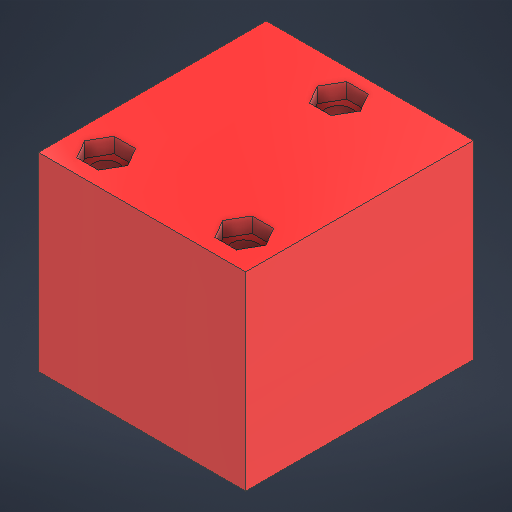
# Autodesk Inventor part: adapter-optical
Saved by Autodesk Inventor 2026.2 (Build 302298000, 298)
## iProperties
Created: 2026-05-22
Part Number: adapter-optical
Material: Generic
Document SubType Name: Modeling
Designer: mayhe
Density: 1 g/cm^3
Appearance: Default
Author: mayhe
Autodesk Inventor part; units mm, degrees
ref_plane "YZ Plane" through (0, 0, 0) normal (1, 0, 0) x (0, 1, 0)
ref_plane "XZ Plane" through (0, 0, 0) normal (0, 1, 0) x (-1, 0, 0)
ref_plane "XY Plane" through (0, 0, 0) normal (0, 0, 1) x (1, 0, 0)
sketch "Sketch1" plane through (0, 0, 0) normal (1, 0, 0) x (0, 1, 0)
  line L0 (13.75, 16.5) -> (-13.75, 16.5)
  line L1 (-13.75, 16.5) -> (-13.75, -16.5)
  line L2 (-13.75, -16.5) -> (13.75, -16.5)
  line L3 (13.75, -16.5) -> (13.75, 16.5)
  line L4 (13.75, 16.5) -> (-13.75, -16.5) construction
  line L5 (-13.75, 16.5) -> (13.75, -16.5) construction
  point P0 (0, 0)
  dimension "d0" = 27.5
  dimension "d1" = 33
  constraints: 12 end point, 2 midpoint, 2 parallel, 1 horizontal, 1 perpendicular
  measures "d0" distance of L2.end L1.end
  measures "d1" distance of L1.end L0.end
extrude "Extrusion1" add sketch "Sketch1" along normal mid plane 30
sketch "Sketch2" plane through (-15, -13.75, -16.5) normal (0, -1, 0) x (1, 0, 0)
  circle A0 centre (15, 4.5) radius 2.25
  line L0 (0, 0) -> (30, 0) projected
  circle A1 centre (25, 28.2) radius 2.25
  circle A2 centre (5, 28.2) radius 2.25
  point P0 (15, 16.5)
  dimension "d4" = 4.5
  dimension "d5" = 4.5
  dimension "d6" = 4.5
  dimension "d7" = 4.5
  dimension "d8" = 23.7
  dimension "d9" = 10
  dimension "d10" = 10
  constraints: 3 centre point, 1 horizontal alignment
  measures "d4" diameter of A0
  measures "d5" distance from line of L0 A0.centre
  measures "d6" diameter of A1
  measures "d7" diameter of A2
  measures "d8" vertical distance of A1.centre A0.centre
  measures "d9" horizontal distance of A0.centre A1.centre
  measures "d10" horizontal distance of A2.centre A0.centre
hole "Hole1" at (0, -13.75, -12) at (-10, -13.75, 11.7) at (10, -13.75, 11.7) direction (0, 1, 0) diameter 3.75 depth 27.5 tip angle 118
sketch "Sketch3" plane through (-15, 13.75, 16.5) normal (0, 1, 0) x (1, 0, 0)
  circle A0 centre (15, 28.5) radius 1.875 projected
  circle A1 centre (25, 4.8) radius 1.875 projected
  circle A2 centre (5, 4.8) radius 1.875 projected
  circle A3 centre (15, 28.5) radius 2.7
  circle A4 centre (5, 4.8) radius 2.7
  circle A5 centre (25, 4.8) radius 2.7
  line L0 (13.4412, 25.8) -> (11.8823, 28.5)
  line L1 (11.8823, 28.5) -> (13.4412, 31.2)
  line L2 (13.4412, 31.2) -> (16.5588, 31.2)
  line L3 (16.5588, 31.2) -> (18.1177, 28.5)
  line L4 (18.1177, 28.5) -> (16.5588, 25.8)
  line L5 (16.5588, 25.8) -> (13.4412, 25.8)
  line L6 (3.4412, 2.1) -> (1.8823, 4.8)
  line L7 (1.8823, 4.8) -> (3.4412, 7.5)
  line L8 (3.4412, 7.5) -> (6.5588, 7.5)
  line L9 (6.5588, 7.5) -> (8.1177, 4.8)
  line L10 (8.1177, 4.8) -> (6.5588, 2.1)
  line L11 (6.5588, 2.1) -> (3.4412, 2.1)
  line L12 (23.4412, 2.1) -> (21.8823, 4.8)
  line L13 (21.8823, 4.8) -> (23.4412, 7.5)
  line L14 (23.4412, 7.5) -> (26.5588, 7.5)
  line L15 (26.5588, 7.5) -> (28.1177, 4.8)
  line L16 (28.1177, 4.8) -> (26.5588, 2.1)
  line L17 (26.5588, 2.1) -> (23.4412, 2.1)
  point P0 (15, 16.5)
  point P1 (15, 25.8)
  point P2 (5, 2.1)
  point P3 (25, 2.1)
  dimension "d18" = 5.4
  dimension "d19" = 5.4
  dimension "d20" = 5.4
  constraints: 36 end point, 6 coincident, 3 midpoint, 3 vertical alignment, 1 point on line, 45 other
extrude "Extrusion2" cut sketch "Sketch3" against normal blind 2.2 contours A0 | A1 | A2 | A3 | A3 L3 L4 | A3 L2 L3 | L4 L5 A3 | A3 L1 L2 | L5 L0 A3 | A3 L0 L1 | A4 | A4 L9 L10 | A4 L8 L9 | L10 L11 A4 | A4 L7 L8 | L11 L6 A4 | A4 L6 L7 | A5 | A5 L15 L16 | A5 L14 L15 | L16 L17 A5 | A5 L13 L14 | L17 L12 A5 | A5 L12 L13
body "Solid1"
